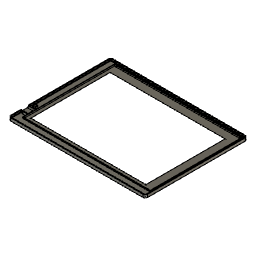
Soldered Inkplate 10 v1.3.0. Top v1.3.2. (Autodesk Fusion 360 design; units mm, degrees)
Autodesk Fusion 360 part; units mm, degrees
sketch "Sketch1" plane through (0, 0, 0) normal (0, 0, 1) x (1, 0, 0)
  line L0 (120.5, 90) -> (-120.5, 90)
  line L1 (-120.5, 90) -> (-120.5, -90)
  line L2 (-120.5, -90) -> (120.5, -90)
  line L3 (120.5, -90) -> (120.5, 90)
  line L4 (120.5, 90) -> (-120.5, -90) construction
  line L5 (-120.5, 90) -> (120.5, -90) construction
  line L6 (101.4, 69.8) -> (-101.4, 69.8)
  line L7 (-101.4, 69.8) -> (-101.4, -69.8)
  line L8 (-101.4, -69.8) -> (101.4, -69.8)
  line L9 (101.4, -69.8) -> (101.4, 69.8)
  line L10 (101.4, 69.8) -> (-101.4, -69.8) construction
  line L11 (-101.4, 69.8) -> (101.4, -69.8) construction
  line L12 (-90, 50) -> (90, 50)
  line L13 (90, 50) -> (90, -50)
  line L14 (90, -50) -> (-90, -50)
  line L15 (-90, -50) -> (-90, 50)
  line L16 (-90, 50) -> (90, -50) construction
  line L17 (90, 50) -> (-90, -50) construction
  dimension "d1" = 241
  dimension "d2" = 180
  dimension "d3" = 20.2
  dimension "d4" = 19.1
  constraint horizontal L0
  constraint perpendicular L0 L1
  constraint parallel L0 L2
  constraint parallel L1 L3
  constraint coincident L4 origin
  constraint coincident L5 origin
  constraint horizontal L6
  constraint perpendicular L6 L7
  constraint parallel L6 L8
  constraint parallel L7 L9
  constraint coincident L10 origin
  constraint coincident L11 origin
  constraint horizontal L12
  constraint perpendicular L12 L13
  constraint parallel L12 L14
  constraint parallel L13 L15
  constraint coincident L16 origin
  constraint coincident L17 origin
  measures "d1" distance of L1.end L2.end
  measures "d2" distance of L0.end L1.end
  measures "d3" distance of L0 L6
  measures "d4" distance of L1 L7
extrude "Extrude1" add sketch "Sketch1" along normal blind 5 contours L0 L1 L2 L3
sketch "Sketch2" plane through (0, 0, 5) normal (0, 0, 1) x (-1, 0, 0)
  line L0 (-101.4, -69.8) -> (-101.4, 69.8)
  line L1 (-101.4, 69.8) -> (101.4, 69.8)
  line L2 (101.4, 69.8) -> (101.4, -69.8)
  line L3 (101.4, -69.8) -> (-101.4, -69.8)
  line L4 (-120.5, 90) -> (-120.5, -90)
  line L5 (-120.5, -90) -> (120.5, -90)
  line L6 (120.5, -90) -> (120.5, 90)
  line L7 (120.5, 90) -> (-120.5, 90)
  line L8 (-119, -88.5) -> (119, -88.5)
  line L9 (119, -88.5) -> (119, 88.5)
  line L10 (119, 88.5) -> (-119, 88.5)
  line L11 (-119, 88.5) -> (-119, -88.5)
  line L12 (-119, -88.5) -> (119, 88.5) construction
  line L13 (119, -88.5) -> (-119, 88.5) construction
  dimension "d7" = 238
  dimension "d8" = 177
  constraint horizontal L8
  constraint perpendicular L8 L9
  constraint parallel L8 L10
  constraint parallel L9 L11
  constraint coincident L12 origin
  constraint coincident L13 origin
  measures "d7" distance of L9.end L10.end
  measures "d8" distance of L8.end L9.end
extrude "Extrude2" cut sketch "Sketch2" against normal blind 3 contours L8 L9 L10 L11
chamfer "Chamfer1" distance 2 distance2 2 4 edges at (0, 69.8, 0) (101.4, 0, 0) (-101.4, 0, 0) (0, -69.8, 0) measured on face at (33.8, 69.8, 0.6667) measured on face at (101.4, -23.2667, 0.6667) measured on face at (-101.4, 23.2667, 0.6667) measured on face at (33.8, -69.8, 1.3333)
fillet "Fillet1" radius 4 4 edges at (-120.5, 90, 2.5) (-120.5, -90, 2.5) (120.5, -90, 2.5) (120.5, 90, 2.5)
sketch "Sketch3" plane through (-120.5, 0, 0) normal (-1, 0, 0) x (0, -1, 0)
  line L0 (86, 0) -> (86, 5)
  line L1 (86, 5) -> (-86, 5)
  line L2 (-86, 5) -> (-86, 0)
  line L3 (-86, 0) -> (86, 0)
  line L4 (90, 0) -> (90, 27.3812) construction
  line L5 (67.848, 25) -> (67.848, -8.2811) construction
  line L6 (67.848, 5) -> (54.848, 5)
  line L7 (54.848, 5) -> (54.848, 2)
  line L8 (54.848, 2) -> (67.848, 2)
  line L9 (67.848, 2) -> (67.848, 5)
  dimension "d15" = 22.152
  dimension "d16" = 13
  dimension "d17" = 3
  constraint perpendicular L1 L4
  constraint perpendicular L3 L5
  constraint horizontal L6
  constraint vertical L7
  constraint horizontal L8
  constraint vertical L9
  constraint coincident L5 L6.start
  constraint coincident L1 L6.start
  measures "d15" distance of L4 L5
  measures "d16" distance of L6.start L6.end
  measures "d17" distance of L6.end L7.end
sketch "Sketch5" plane through (0, 0, 2) normal (0, 0, 1) x (-1, 0, 0)
  line L0 (101.4, 69.8) -> (101.4, -69.8)
  line L1 (101.4, -69.8) -> (-101.4, -69.8)
  line L2 (-101.4, -69.8) -> (-101.4, 69.8)
  line L3 (-101.4, 69.8) -> (101.4, 69.8)
  line L4 (-119, 88.5) -> (-119, -88.5)
  line L5 (-119, -88.5) -> (119, -88.5)
  line L6 (119, -88.5) -> (119, 88.5)
  line L7 (119, 88.5) -> (-119, 88.5)
  line L8 (111, 67.848) -> (141, 67.848) construction
  line L9 (116.5, 90) -> (-116.5, 90) construction
  line L10 (112.5407, 54.848) -> (136.5407, 54.848) construction
  line L11 (109.2, 77) -> (109.2, 48) construction
  line L12 (111, 69.848) -> (124, 69.848) construction
  line L13 (112, 52.848) -> (123, 52.848) construction
  line L14 (115.8, 52.848) -> (109.2, 52.848)
  line L15 (109.2, 52.848) -> (109.2, 69.848)
  line L16 (109.2, 69.848) -> (115.8, 69.848)
  line L17 (115.8, 69.848) -> (115.8, 54.848)
  line L18 (119, 54.848) -> (115.8, 54.848)
  line L19 (115.8, 52.848) -> (119, 52.848)
  line L20 (119, 52.848) -> (119, 54.848)
  line L21 (115.8, 77) -> (115.8, 54.848) construction
  line L22 (115.8, 52.848) -> (115.8, 49) construction
  dimension "d22" = 22.152
  dimension "d23" = 13
  dimension "d24" = 9.8
  dimension "d25" = 3.2
  dimension "d26" = 2
  dimension "d27" = 2
  constraint horizontal L8
  constraint perpendicular L6 L10
  constraint vertical L11
  constraint vertical L21
  constraint horizontal L12
  constraint horizontal L13
  constraint horizontal L14
  constraint vertical L15
  constraint horizontal L16
  constraint vertical L17
  constraint coincident L13 L14.start
  constraint coincident L14.start L21
  constraint coincident L11 L14.end
  constraint coincident L12 L16.end
  constraint horizontal L18
  constraint horizontal L19
  constraint vertical L20
  constraint coincident L10 L18.start
  constraint coincident L6 L18.start
  constraint collinear L21 L22
  measures "d22" distance of L8 L9
  measures "d23" distance of L8 L10
  measures "d24" distance of L6 L11
  measures "d25" distance of L6 L21
  measures "d26" distance of L8 L12
  measures "d27" distance of L10 L13
extrude "Extrude4" add sketch "Sketch5" along normal blind 3 contours L6 L14 L15 L16 L17 L18 L19 L20
sketch "Sketch6" plane through (0, 0, 2) normal (0, 0, 1) x (-1, 0, 0)
  line L0 (115.8, 69.848) -> (115.8, 54.848)
  line L1 (119, 52.848) -> (109.2, 52.848)
  line L2 (109.2, 52.848) -> (109.2, 69.848)
  line L3 (109.2, 69.848) -> (115.8, 69.848)
  line L4 (101.4, 69.8) -> (101.4, -69.8)
  line L5 (101.4, -69.8) -> (-101.4, -69.8)
  line L6 (-101.4, -69.8) -> (-101.4, 69.8)
  line L7 (-101.4, 69.8) -> (101.4, 69.8)
  line L8 (-119, 88.5) -> (-119, -88.5)
  line L9 (-119, -88.5) -> (119, -88.5)
  line L10 (119, 54.848) -> (119, 88.5)
  line L11 (119, 88.5) -> (-119, 88.5)
  line L12 (109.2, 69.848) -> (109.2, 76.7) construction
  line L13 (97, 76.7) -> (115, 76.7) construction
  line L14 (109.2, 76.7) -> (107.2, 76.7)
  line L15 (107.2, 74.7) -> (107.2, -83.3)
  line L16 (109.2, -85.3) -> (109.2, 76.7)
  line L17 (107.2, 76.7) -> (-116, 76.7)
  line L18 (-116, 76.7) -> (-116, 71.5114)
  line L19 (-114, 74.7) -> (107.2, 74.7)
  line L20 (-114, 74.7) -> (-114, -83.3)
  line L21 (-112.7, -85.3) -> (-116, -85.3)
  line L22 (-116, -85.3) -> (-116, 71.5114)
  line L23 (-116, -85.3) -> (109.2, -85.3)
  line L24 (107.2, -83.3) -> (-114, -83.3)
  line L25 (-116, -81.7) -> (-116, -85.3)
  line L26 (107.2, 88.5464) -> (107.2, 76.7) construction
  line L27 (107.2, 74.7) -> (107.2, -80.0928) construction
  line L28 (116.5, 90) -> (-116.5, 90)
  line L29 (-116.5, -90) -> (116.5, -90)
  line L30 (-120.5, 86) -> (-120.5, -86)
  line L31 (115.8, 54.848) -> (119, 54.848)
  line L32 (119, -88.5) -> (119, 52.848)
  dimension "d30" = 2
  dimension "d36" = 2
  dimension "d42" = 2
  dimension "d43" = 2
  dimension "d51" = 15.3
  dimension "d52" = 6.7
  dimension "d53" = 6.5
  constraint vertical L26
  constraint coincident L2.end L3.start
  constraint perpendicular L3 L12
  constraint perpendicular L13 L26
  constraint coincident L12.end L13
  constraint horizontal L14
  constraint vertical L15
  constraint vertical L16
  constraint horizontal L17
  constraint vertical L18
  constraint horizontal L19
  constraint vertical L20
  constraint horizontal L21
  constraint vertical L22
  constraint horizontal L23
  constraint horizontal L24
  constraint vertical L25
  constraint collinear L26 L27
  constraint coincident L16.start L23
  measures "d30" distance of L2 L26
  measures "d36" distance of L14.end L15.start
  measures "d42" distance of L20 L22
  measures "d43" distance of L23 L24
  measures "d51" distance of L19 L28
  measures "d52" distance of L24 L29
  measures "d53" distance of L20 L30
extrude "Extrude5" add sketch "Sketch6" along normal blind 1.2 contours L2 L14 L16 L17 L18 L21 L22 L23 L25
extrude "Extrude3" cut sketch "Sketch3" against normal blind 11.3 contours L1 L6 L7 L8 L9
fillet "Fillet2" radius 2 5 edges at (-114.85, -54.848, 2) (-119.75, -67.848, 2) (-112.5, -67.848, 2) (-114.85, -54.848, 2) (-109.2, -61.348, 2)
ref_plane "WorkPlane1" through (-0.75, 0, 2.5) normal (0, 0, 1) x (1, 0, 0)
sketch "Sketch7" plane through (-1, 0, 2.5) normal (0, 0, 1) x (1, 0, 0)
  line L0 (-123, -52.848) -> (-103, -52.848) construction
  line L1 (-118, 99.3909) -> (-118, -54.5) construction
  line L2 (-118, -52.848) -> (-117, -52.848)
  line L3 (-117, -52.848) -> (-117, 86.5)
  line L4 (-117, 88.5) -> (-118, 88.5)
  line L5 (-118, 85) -> (-118, -52.848)
  line L6 (-114.5, 88.5) -> (120, 88.5)
  line L7 (120, 88.5) -> (120, 87.5)
  line L8 (118, 87.5) -> (-116, 87.5)
  line L9 (-118, 87.5) -> (-118, 88.5)
  line L10 (120, 88.5) -> (120, -88.5)
  line L11 (120, 88.5) -> (119, 88.5)
  line L12 (119, 86.5) -> (119, -86.5)
  line L13 (119, -88.5) -> (120, -88.5)
  line L14 (120, -88.5) -> (120, 88.5)
  arc A0 (-116, 87.5) -> (-117, 86.5) centre (-116, 86.5) ccw
  line L15 (-118, 88.5) -> (-118, 84.5)
  line L16 (-118, 88.5) -> (-114.5, 88.5)
  arc A1 (119, 86.5) -> (118, 87.5) centre (118, 86.5) ccw
  line L17 (120, -88.5) -> (-118, -88.5)
  line L18 (-118, -88.5) -> (-118, -87.5)
  line L19 (-116, -87.5) -> (118, -87.5)
  line L20 (120, -87.5) -> (120, -88.5)
  line L21 (-118, -88.5) -> (-118, -67.848)
  line L22 (-118, -88.5) -> (-117, -88.5)
  line L23 (-117, -86.5) -> (-117, -69.848)
  line L24 (-117, -69.848) -> (-118, -69.848)
  line L25 (-118, -69.848) -> (-118, -88.5)
  line L26 (-114.8, -69.848) -> (-119.2313, -69.848) construction
  arc A2 (-117, -86.5) -> (-116, -87.5) centre (-116, -86.5) ccw
  arc A3 (118, -87.5) -> (119, -86.5) centre (118, -86.5) ccw
  line L27 (-118, -88.5) -> (-118, -67.848)
  line L28 (-118, -52.848) -> (-118, 88.5)
  point P0 (-114.8, -52.848)
  point P1 (-114.8, -69.848)
  dimension "d46" = 1
  dimension "d56" = 1
  dimension "d57" = 1
  dimension "d59" = 1
  dimension "d64" = 1
  dimension "d65" = 1
  dimension "d66" = 1
  dimension "d67" = 1
  dimension "d68" = 1
  constraint horizontal L0
  constraint coincident L0 P0
  constraint perpendicular L0 L1
  constraint horizontal L2
  constraint vertical L3
  constraint horizontal L4
  constraint vertical L5
  constraint coincident L1 L2.start
  constraint coincident L0 L2.start
  constraint horizontal L6
  constraint vertical L7
  constraint horizontal L8
  constraint vertical L9
  constraint coincident L7.end L10
  constraint horizontal L11
  constraint vertical L12
  constraint horizontal L13
  constraint vertical L14
  constraint coincident L6.end L7.start
  constraint coincident L10.end L13.end
  constraint coincident L4.end L6
  constraint coincident L9.start L8
  constraint coincident L4.start L3
  constraint tangent L8 A0
  constraint tangent L3 A0
  constraint coincident L1 L15.end
  constraint coincident L7.end L8
  constraint coincident L11.end L12
  constraint tangent L8 A1
  constraint tangent L12 A1
  constraint horizontal L17
  constraint vertical L18
  constraint horizontal L19
  constraint vertical L20
  constraint coincident L18.end L21
  constraint horizontal L22
  constraint vertical L23
  constraint horizontal L24
  constraint vertical L25
  constraint coincident L17.end L18.start
  constraint horizontal L26
  constraint coincident L23.end L26
  constraint coincident L22.end L23
  constraint coincident L18.end L19
  constraint tangent L23 A2
  constraint tangent L19 A2
  constraint coincident L13.start L12
  constraint coincident L20.start L19
  constraint tangent L12 A3
  constraint tangent L19 A3
  measures "d46" distance of L2.start L2.end
  measures "d56" distance of L4.end L9.start
  measures "d57" distance of L6.end L11.end
  measures "d59" radius of A0
  measures "d64" radius of A1
  measures "d65" distance of L10.end L20.start
  measures "d66" distance of L17.end L22.end
  measures "d67" radius of A2
  measures "d68" radius of A3
extrude "Extrude6" add sketch "Sketch7" along normal blind 2.5
chamfer "Chamfer2" distance 1.5 distance2 1.5 9 edges at (-118, 16.826, 2.5) (-117.7071, 87.2071, 2.5) (0, 87.5, 2.5) (117.7071, 87.2071, 2.5) (118, 0, 2.5) (117.7071, -87.2071, 2.5) (0, -87.5, 2.5) (-117.7071, -87.2071, 2.5) (-118, -78.174, 2.5) measured on face at (-118, -6.3987, 3.3333) measured on face at (-39, -88.1667, 2.5) measured on face at (-39, -88.1667, 2.5) measured on face at (-39, -88.1667, 2.5) measured on face at (118, 28.8333, 3.3333) measured on face at (-39, -88.1667, 2.5) measured on face at (-39, -88.1667, 2.5) measured on face at (-39, -88.1667, 2.5) measured on face at (-118, -80.9493, 4.1667)
sketch "Sketch9" plane through (0, 0, 2) normal (0, 0, 1) x (-1, 0, 0)
  line L0 (120.5, 65.848) -> (119, 65.848)
  line L1 (119, 65.848) -> (119, 88.5)
  line L2 (119, 52.848) -> (109.2, 52.848)
  line L3 (109.2, 52.848) -> (109.2, -85.3)
  line L4 (109.2, -85.3) -> (-116, -85.3)
  line L5 (-116, -85.3) -> (-116, 76.7)
  line L6 (-116, 76.7) -> (109.2, 76.7)
  line L7 (109.2, 76.7) -> (109.2, 69.848)
  line L8 (109.2, 69.848) -> (115.8, 69.848)
  line L9 (115.8, 69.848) -> (115.8, 65.848)
  line L10 (115.8, 65.848) -> (111.033, 65.848)
  line L11 (111.033, 65.848) -> (111.033, 56.848)
  line L12 (111.033, 56.848) -> (120.5, 56.848)
  line L13 (120.5, 56.848) -> (120.5, 65.848)
  line L14 (115.8, 69.848) -> (119, 69.848)
  line L15 (119, 88.5) -> (-119, 88.5)
  line L16 (-119, 88.5) -> (-119, -88.5)
  line L17 (-119, -88.5) -> (119, -88.5)
  line L18 (119, -88.5) -> (119, 52.848)
  constraint coincident L8.end L9.start
  constraint coincident L1 L14.end
  constraint perpendicular L1 L14
extrude "Extrude11" cut sketch "Sketch9" against normal blind 0.5 contours L1 L2 L3 L4 L5 L6 L7 L8 L14 L15 L16 L17 L18
chamfer "Chamfer5" distance 1 angle 45 9 edges at (-118, -78.174, 5) (-118, 16.826, 5) (-117.7071, 87.2071, 5) (0, 87.5, 5) (117.7071, 87.2071, 5) (118, 0, 5) (117.7071, -87.2071, 5) (0, -87.5, 5) (-117.7071, -87.2071, 5)
chamfer "Chamfer6" distance 1.2 angle 45 4 edges at (3.4, -74.7, 3.2) (-107.2, 4.3, 3.2) (114, 4.3, 3.2) (3.4, 83.3, 3.2)
sketch "Sketch10" plane through (0, 0, 1.5) normal (0, 0, 1) x (-1, 0, 0)
  line L0 (119, -88.5) -> (119, 52.848)
  line L1 (119, 52.848) -> (109.2, 52.848)
  line L2 (109.2, 52.848) -> (109.2, -85.3)
  line L3 (109.2, -85.3) -> (-116, -85.3)
  line L4 (-116, -85.3) -> (-116, 76.7)
  line L5 (-116, 76.7) -> (109.2, 76.7)
  line L6 (109.2, 76.7) -> (109.2, 69.848)
  line L7 (109.2, 69.848) -> (119, 69.848)
  line L8 (119, 69.848) -> (119, 88.5)
  line L9 (119, 88.5) -> (-119, 88.5)
  line L10 (-119, 88.5) -> (-119, -88.5)
  line L11 (-119, -88.5) -> (119, -88.5)
  line L12 (111, 52.848) -> (114.5, 52.848)
  line L13 (114.5, 52.848) -> (114.5, 47.848)
  line L14 (114.5, 47.848) -> (111, 47.848)
  line L15 (111, 47.848) -> (111, 52.848)
  line L16 (120.5, -86) -> (120.5, 54.848)
  dimension "d84" = 3.5
  dimension "d85" = 5
  dimension "d86" = 6
  constraint horizontal L12
  constraint vertical L13
  constraint horizontal L14
  constraint vertical L15
  constraint coincident L1 L12.start
  measures "d84" distance of L12.start L12.end
  measures "d85" distance of L12.start L14.end
  measures "d86" distance of L13 L16
extrude "Extrude12" add sketch "Sketch10" along normal blind 4.1 contours L1 L12 L13 L14 L15
chamfer "Chamfer7" distance 0.5 angle 45 1 edges at (-111, -50.348, 5.6)
